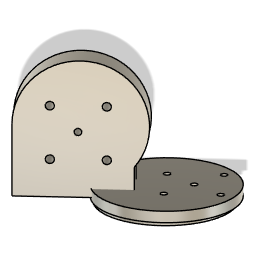
rotating part of a mechanical hand (Autodesk Fusion 360 design; units mm, degrees)
part number: 2025-07-26-20-09-52-917
Autodesk Fusion 360 part; units mm, degrees
sketch "Sketch1" plane through (0, 0, 0) normal (0, 0, 1) x (1, 0, 0)
  circle A0 centre (-0.7975, 0) radius 50
  dimension "d1" = 100
  measures "d1" diameter of A0
extrude "Extrude1" add sketch "Sketch1" along normal blind 10 makes body 1
sketch "Sketch2" plane through (0, 0, 0) normal (0, 0, -1) x (1, 0, 0)
  circle A0 centre (-0.7975, 0) radius 50
  circle A1 centre (0, 0) radius 47.5
  dimension "d4" = 95
  constraint coincident A1.centre origin
  measures "d4" diameter of A1
extrude "Extrude2" cut sketch "Sketch2" against normal blind 3 contours A1 bodies 1
extrude "Extrude3" add 1 faces at (-13.9218, -0.7502, 3) along direction (0, 0, -1) blind 3 on bodies 1 bodies 1
extrude "Extrude4" add sketch "Sketch2" along normal blind 3 contours A1 bodies 1
extrude "Extrude5" cut 1 faces at (-14.3493, -2.484, 10) along direction (0, 0, -1) blind 2 on bodies 1 bodies 1
sketch "Sketch3" plane through (0, 0, 0) normal (0, 1, 0) x (1, 0, 0)
  line L0 (20, -10) -> (100, -10)
  line L1 (100, -10) -> (100, -60)
  arc A0 (20, -31.7157) -> (100, -60) centre (55, -60) ccw
  line L2 (20, -31.7157) -> (20, -10)
  dimension "d13" = 80
  dimension "d14" = 50
  dimension "d15" = 45
  dimension "d16" = 20
  dimension "d17" = 60
  constraint horizontal L0
  constraint perpendicular L0 L1
  constraint tangent L1 A0
  constraint vertical L2
  measures "d13" distance of L0.start L0.end
  measures "d14" distance of L0.end L1.end
  measures "d15" radius of A0
  measures "d16" horizontal distance of L0.start origin
  measures "d17" vertical distance of A0.centre origin
extrude "Extrude6" add sketch "Sketch3" along normal mid plane 20 separate body makes body 2
move_body "Move1" bodies 2 to x (1, 0, 0) y (0, 1, 0) z (0, 0, 1) at (-0.2318, 0.064, -8.407)
sketch "Sketch4" plane through (0, 10.064, 0) normal (0, 1, 0) x (-1, 0, 0)
  arc A0 (-19.7682, 23.3087) -> (-99.7682, 51.593) centre (-54.7682, 51.593) ccw
  line L0 (-99.7682, 51.593) -> (-99.7682, 1.593)
  line L1 (-99.7682, 1.593) -> (-19.7682, 1.593)
  line L2 (-19.7682, 1.593) -> (-19.7682, 23.3087)
  line L3 (-75, 65) -> (-37.756, 65)
  line L4 (-37.756, 65) -> (-37.756, 27.756)
  line L5 (-37.756, 27.756) -> (-75, 27.756)
  line L6 (-75, 27.756) -> (-75, 65)
  dimension "d20" = 37.244
  dimension "d21" = 37.244
  dimension "d22" = 17.0122
  constraint horizontal L3
  constraint vertical L4
  constraint horizontal L5
  constraint vertical L6
  measures "d20" distance of L3.start L3.end
  measures "d21" distance of L3.start L5.end
  measures "d22" distance of A0.centre L4
sketch "Sketch5" plane through (0, 10.064, 0) normal (0, 1, 0) x (-1, 0, 0)
  arc A0 (-19.7682, 23.3087) -> (-99.7682, 51.593) centre (-54.7682, 51.593) ccw
  line L0 (-99.7682, 51.593) -> (-99.7682, 1.593)
  line L1 (-99.7682, 1.593) -> (-19.7682, 1.593)
  line L2 (-19.7682, 1.593) -> (-19.7682, 23.3087)
  line L3 (-75, 65) -> (-38, 28)
  line L4 (-38, 65) -> (-75, 28)
hole "Hole2" at (75, 10.064, 65) at (37.756, 10.064, 65) at (75, 10.064, 27.756) at (37.756, 10.064, 27.756) direction (0, -1, 0) diameter 6 end through all bodies 2
sketch "Sketch6" plane through (0, 10.064, 0) normal (0, 1, 0) x (-1, 0, 0)
hole "Hole3" at (56.6237, 10.064, 47.0814) direction (0, -1, 0) diameter 5 end through all bodies 2
sketch "Sketch7" plane through (0, 0, 8) normal (0, 0, 1) x (-1, 0, 0)
  circle A0 centre (0.7975, 0) radius 50
  line L0 (37.1703, -17.1797) -> (-0.0737, -17.1797)
  line L1 (-0.0737, -17.1797) -> (-0.0737, 20.0643)
  line L2 (-0.0737, 20.0643) -> (37.1703, 20.0643)
  line L3 (37.1703, 20.0643) -> (37.1703, -17.1797)
  point P0 (0.7975, 0)
  dimension "d29" = 37.244
  dimension "d30" = 37.244
  constraint horizontal L0
  constraint vertical L1
  constraint horizontal L2
  constraint vertical L3
  measures "d29" distance of L0.start L0.end
  measures "d30" distance of L0.start L2.end
hole "Hole4" at (-37.1703, 17.1797, 8) at (0.0737, 17.1797, 8) at (-37.1703, -20.0643, 8) at (0.0737, -20.0643, 8) direction (0, 0, -1) diameter 5 end through all bodies 1
sketch "Sketch8" plane through (0, -9.936, 0) normal (0, -1, 0) x (1, 0, 0)
  circle A0 centre (56.6237, 47.0814) radius 2.5
  circle A1 centre (75, 27.756) radius 3
  circle A2 centre (75, 65) radius 3
  circle A3 centre (37.756, 65) radius 3
  circle A4 centre (37.756, 27.756) radius 3
  arc A5 (99.7682, 51.593) -> (19.7682, 23.3087) centre (54.7682, 51.593) ccw
  line L0 (19.7682, 23.3087) -> (19.7682, 1.593)
  line L1 (19.7682, 1.593) -> (99.7682, 1.593)
  line L2 (99.7682, 1.593) -> (99.7682, 51.593)
sketch "Sketch9" plane through (0, 10.064, 0) normal (0, 1, 0) x (-1, 0, 0)
  circle A0 centre (-56.6237, 47.0814) radius 2.5
  circle A1 centre (-75, 27.756) radius 3
  circle A2 centre (-75, 65) radius 3
  circle A3 centre (-37.756, 65) radius 3
  circle A4 centre (-37.756, 27.756) radius 3
  arc A5 (-19.7682, 23.3087) -> (-99.7682, 51.593) centre (-54.7682, 51.593) ccw
  line L0 (-99.7682, 51.593) -> (-99.7682, 1.593)
  line L1 (-99.7682, 1.593) -> (-19.7682, 1.593)
  line L2 (-19.7682, 1.593) -> (-19.7682, 23.3087)
sketch "Sketch10" plane through (0, 0, 8) normal (0, 0, 1) x (-1, 0, 0)
  circle A0 centre (37.1703, 20.0643) radius 2.5
  circle A1 centre (37.1703, -17.1797) radius 2.5
  circle A2 centre (-0.0737, -17.1797) radius 2.5
  circle A3 centre (-0.0737, 20.0643) radius 2.5
  circle A4 centre (0.7975, 0) radius 50
  line L0 (37.1703, -17.1797) -> (-0.0737, 20.0643)
  line L1 (-0.0737, -17.1797) -> (37.1703, 20.0643)
  constraint coincident A1.centre L0.start
  constraint coincident A3.centre L0.end
  constraint coincident A2.centre L1.start
  constraint coincident A0.centre L1.end
hole "Hole5" at (-18.7289, -1.1433, 8) direction (0, 0, -1) diameter 5 end through all bodies 1
hole "Hole1" [suppressed]
